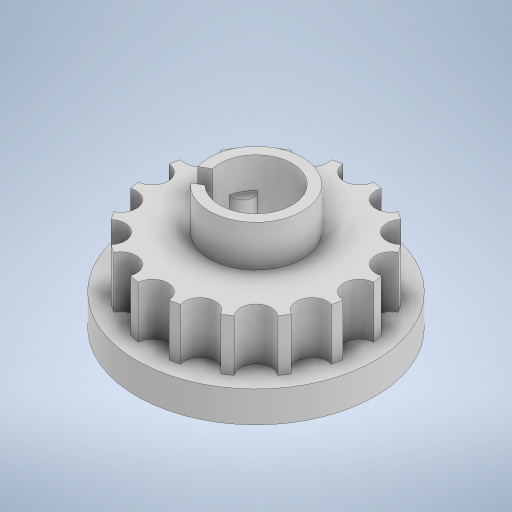
# Autodesk Inventor part: вращалка
Saved by Autodesk Inventor 2023 (Build 270158000, 158)
## iProperties
Created: 2023-04-09
Part Number: вращалка
Material: Типовые
Document SubType Name: Modeling
Designer: deryu
Density: 1 g/cm^3
Appearance: По умолчанию
Author: deryu
Autodesk Inventor part; units mm, degrees
ref_plane "YZ Plane" through (0, 0, 0) normal (1, 0, 0) x (0, 1, 0)
ref_plane "XZ Plane" through (0, 0, 0) normal (0, 1, 0) x (-1, 0, 0)
ref_plane "XY Plane" through (0, 0, 0) normal (0, 0, 1) x (1, 0, 0)
sketch "Эскиз1" plane through (0, 0, 0) normal (0, 1, 0) x (-1, 0, 0)
  circle A0 centre (0, 0) radius 11.5
  circle A1 centre (0, 0) radius 8.5
  dimension "d0" = 23
  dimension "d1" = 17
  constraints: 2 centre point, 2 coincident
  measures "d0" diameter of A0
  measures "d1" diameter of A1
extrude "Выдавливание1" add sketch "Эскиз1" along normal blind 3
sketch "Эскиз2" plane through (0, 3, 0) normal (0, 1, 0) x (1, 0, 0)
  circle A0 centre (0, 0) radius 10
  circle A1 centre (-10, 0) radius 1.5
  circle A2 centre (-9.2388, -3.8268) radius 1.5
  circle A3 centre (-7.0711, -7.0711) radius 1.5
  circle A4 centre (-3.8268, -9.2388) radius 1.5
  circle A5 centre (0, -10) radius 1.5
  circle A6 centre (3.8268, -9.2388) radius 1.5
  circle A7 centre (7.0711, -7.0711) radius 1.5
  circle A8 centre (9.2388, -3.8268) radius 1.5
  circle A9 centre (10, 0) radius 1.5
  circle A10 centre (9.2388, 3.8268) radius 1.5
  circle A11 centre (7.0711, 7.0711) radius 1.5
  circle A12 centre (3.8268, 9.2388) radius 1.5
  circle A13 centre (0, 10) radius 1.5
  circle A14 centre (-3.8268, 9.2388) radius 1.5
  circle A15 centre (-7.0711, 7.0711) radius 1.5
  circle A16 centre (-9.2388, 3.8268) radius 1.5
  point P0 (-8.5625, 5.1657)
  point P1 (-9.7073, 2.4019)
  point P2 (-9.8875, 1.4958)
  point P3 (-9.8875, -1.4958)
  point P4 (-9.7073, -2.4019)
  point P5 (-8.5625, -5.1657)
  point P6 (-8.0492, -5.9338)
  point P7 (-5.9338, -8.0492)
  point P8 (-5.1657, -8.5625)
  point P9 (-2.4019, -9.7073)
  point P10 (-1.4958, -9.8875)
  point P11 (1.4958, -9.8875)
  point P12 (2.4019, -9.7073)
  point P13 (5.1657, -8.5625)
  point P14 (5.9338, -8.0492)
  point P15 (8.0492, -5.9338)
  point P16 (8.5625, -5.1657)
  point P17 (9.7073, -2.4019)
  point P18 (9.8875, -1.4958)
  point P19 (9.8875, 1.4958)
  point P20 (9.7073, 2.4019)
  point P21 (8.5625, 5.1657)
  point P22 (8.0492, 5.9338)
  point P23 (5.9338, 8.0492)
  point P24 (5.1657, 8.5625)
  point P25 (2.4019, 9.7073)
  point P26 (1.4958, 9.8875)
  point P27 (-1.4958, 9.8875)
  point P28 (-2.4019, 9.7073)
  point P29 (-5.1657, 8.5625)
  point P30 (-5.9338, 8.0492)
  point P31 (-8.0492, 5.9338)
  dimension "d4" = 20
  dimension "d5" = 3
  dimension "d8" = 360
  constraints: 16 centre point, 1 coincident, 36 other
  measures "d5" diameter of A1
extrude "Выдавливание2" add sketch "Эскиз2" along normal blind 5 contours A9 A0 A8 A7 A6 A5 A4 A3 A2 A1 A16 A15 A14 A13 A12 A11 A10
sketch "Эскиз3" plane through (0, 8, 0) normal (0, 1, 0) x (1, 0, 0)
  circle A0 centre (0, 0) radius 4.5
  circle A1 centre (0, 0) radius 3.5
  dimension "d12" = 9
  dimension "d13" = 7
  constraints: 2 centre point, 2 coincident
  measures "d12" diameter of A0
  measures "d13" diameter of A1
extrude "Выдавливание3" add sketch "Эскиз3" along normal blind 4
sketch "Эскиз4" plane through (0, 8, 0) normal (0, 1, 0) x (1, 0, 0)
  circle A0 centre (0, 0) radius 3.5
  constraints: 1 centre point, 1 coincident
extrude "Выдавливание4" cut sketch "Эскиз4" against normal through all
sketch "Эскиз5" plane through (0, 3, 0) normal (0, -1, 0) x (1, 0, 0)
  circle A0 centre (0, 0) radius 3.5
  circle A1 centre (0, 0) radius 3.5 projected
  circle A2 centre (0, 3.5) radius 1
  circle A3 centre (-3.0311, -1.75) radius 1
  circle A4 centre (3.0311, -1.75) radius 1
  point P0 (-0.9897, 3.3571)
  point P1 (0.9897, 3.3571)
  point P2 (3.4022, -0.8214)
  point P3 (2.4125, -2.5357)
  point P4 (-3.4022, -0.8214)
  point P5 (-2.4125, -2.5357)
  dimension "d18" = 2
  dimension "d21" = 360
  constraints: 4 centre point, 1 coincident, 1 vertical alignment, 8 other
  measures "d18" diameter of A2
extrude "Выдавливание5" add sketch "Эскиз5" against normal blind 6 contours A2 A0 | A0 A4 | A3 A0 picked at (0, 3.156) picked at (2.7332, -1.578) picked at (-2.7274, -1.5885)
sketch "Эскиз6" plane through (0, 12, 0) normal (0, 1, 0) x (1, 0, 0)
  arc A0 (2.4125, 2.5357) -> (3.4022, 0.8214) centre (3.0311, 1.75) ccw projected
  line L0 (0, 0) -> (3.0311, 1.75)
  line L1 (0, 0) -> (-4.9072, -2.8332)
  line L2 (-4.6871, -3.8608) -> (-2.1071, -2.3712)
  line L3 (-2.1071, -2.3712) -> (-3.1071, -0.6392)
  line L4 (-3.1071, -0.6392) -> (-5.6871, -2.1288)
  line L5 (-5.6871, -2.1288) -> (-4.6871, -3.8608)
  circle A1 centre (0, 0) radius 4.5 projected
  line L6 (-4.6871, -3.8608) -> (-3.1071, -0.6392) construction
  line L7 (-2.1071, -2.3712) -> (-5.6871, -2.1288) construction
  point P0 (-3.8971, -2.25)
  dimension "d25" = 2
  constraints: 16 end point, 2 midpoint, 2 parallel, 1 perpendicular, 1 point on line, 2 other
  measures "d25" distance of L3.end L2.end
extrude "Выдавливание6" cut sketch "Эскиз6" against normal blind 4 contours L3 L2 A1 L1 | L1 A1 L4 L3 | A1 L2 L5 L4
